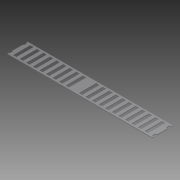
# Autodesk Inventor part: Wing
Saved by Autodesk Inventor 2013 (Build 170138000, 138)
## iProperties
Created: 2013-01-27
Part Number: Wing
Material: Polycarbonate, Clear
Document SubType Name: Modeling
Designer: Andrew Toennies
Density: 1.2 g/cm^3
Mass: 103.546 g
Surface Area: 686.087 cm^2
Volume: 86.2881 cm^3
Author: Andrew Toennies
Autodesk Inventor part; units mm, degrees
ref_plane "YZ Plane" through (0, 0, 0) normal (1, 0, 0) x (0, 1, 0)
ref_plane "XZ Plane" through (0, 0, 0) normal (0, 1, 0) x (-1, 0, 0)
ref_plane "XY Plane" through (0, 0, 0) normal (0, 0, 1) x (1, 0, 0)
sketch "Sketch1" plane through (0, 0, 0) normal (0, 1, 0) x (-1, 0, 0)
  line L0 (0, 0) -> (558.8, 0)
  line L1 (558.8, 0) -> (558.8, 79.375)
  line L2 (558.8, 79.375) -> (0, 79.375)
  line L3 (0, 79.375) -> (0, 0)
  dimension "d0" = 79.375
  dimension "d1" = 558.8
  constraints: 8 end point, 2 parallel, 1 horizontal, 1 perpendicular
  measures "d0" distance of L2.end L0.start
  measures "d1" distance of L1.end L2.end
extrude "Extrusion1" add sketch "Sketch1" along normal blind 3.175
sketch "Sketch3" plane through (-558.8, 0, 0) normal (-1, 0, 0) x (0, 0, 1)
  line L0 (0, 0) -> (79.375, 0) projected
  line L1 (79.375, 0) -> (79.375, 3.175) projected
  line L2 (0, 3.175) -> (79.375, 3.175) projected
  line L3 (0, 0) -> (0, 3.175) projected
  line L4 (73.025, 3.175) -> (73.025, 0)
  line L5 (60.325, 0) -> (60.325, 3.175)
  line L6 (19.05, 0) -> (19.05, 3.175)
  line L7 (6.35, 0) -> (6.35, 3.175)
  dimension "d4" = 12.7
  dimension "d5" = 6.35
  dimension "d6" = 12.7
  dimension "d7" = 6.35
  constraints: 8 end point, 8 point on line, 4 perpendicular
  measures "d4" distance between parallel lines of L5 L4
  measures "d5" distance between parallel lines of L1 L4
  measures "d6" distance between parallel lines of L6 L7
  measures "d7" distance between parallel lines of L3 L7
extrude "Extrusion2" cut sketch "Sketch3" against normal blind 3.175 contours L7 L2 L6 L0 | L5 L2 L4 L0
sketch "Sketch4" plane through (0, 0, 79.375) normal (1, 0, 0) x (0, 0, -1)
  line L0 (19.05, 3.175) -> (6.35, 3.175) projected
  line L1 (19.05, 0) -> (19.05, 3.175) projected
  line L2 (6.35, 0) -> (19.05, 0) projected
  line L3 (6.35, 3.175) -> (6.35, 0) projected
  line L4 (60.325, 3.175) -> (60.325, 0) projected
  line L5 (73.025, 3.175) -> (60.325, 3.175) projected
  line L6 (73.025, 0) -> (73.025, 3.175) projected
  line L7 (60.325, 0) -> (73.025, 0) projected
extrude "Extrusion3" cut sketch "Sketch4" against normal blind 6.35
sketch "Sketch5" plane through (0, 0, 0) normal (0, -1, 0) x (1, 0, 0)
  line L0 (-558.8, 79.375) -> (0, 79.375) projected
  line L1 (-558.8, 19.05) -> (-558.8, 60.325) projected
  line L2 (0, 0) -> (-558.8, 0) projected
  line L3 (-542.925, 73.025) -> (-542.925, 6.35)
  line L4 (-542.925, 6.35) -> (-530.225, 6.35)
  line L5 (-542.925, 73.025) -> (-530.225, 73.025)
  line L6 (-530.225, 73.025) -> (-530.225, 6.35)
  line L7 (-517.525, 73.025) -> (-517.525, 6.35)
  line L8 (-517.525, 6.35) -> (-504.825, 6.35)
  line L9 (-517.525, 73.025) -> (-504.825, 73.025)
  line L10 (-504.825, 73.025) -> (-504.825, 6.35)
  line L11 (-492.125, 73.025) -> (-492.125, 6.35)
  line L12 (-492.125, 6.35) -> (-479.425, 6.35)
  line L13 (-492.125, 73.025) -> (-479.425, 73.025)
  line L14 (-479.425, 73.025) -> (-479.425, 6.35)
  line L15 (-466.725, 73.025) -> (-466.725, 6.35)
  line L16 (-466.725, 6.35) -> (-454.025, 6.35)
  line L17 (-466.725, 73.025) -> (-454.025, 73.025)
  line L18 (-454.025, 73.025) -> (-454.025, 6.35)
  line L19 (-441.325, 73.025) -> (-441.325, 6.35)
  line L20 (-441.325, 6.35) -> (-428.625, 6.35)
  line L21 (-441.325, 73.025) -> (-428.625, 73.025)
  line L22 (-428.625, 73.025) -> (-428.625, 6.35)
  line L23 (-415.925, 73.025) -> (-415.925, 6.35)
  line L24 (-415.925, 6.35) -> (-403.225, 6.35)
  line L25 (-415.925, 73.025) -> (-403.225, 73.025)
  line L26 (-403.225, 73.025) -> (-403.225, 6.35)
  line L27 (-390.525, 73.025) -> (-390.525, 6.35)
  line L28 (-390.525, 6.35) -> (-377.825, 6.35)
  line L29 (-390.525, 73.025) -> (-377.825, 73.025)
  line L30 (-377.825, 73.025) -> (-377.825, 6.35)
  line L31 (-365.125, 73.025) -> (-365.125, 6.35)
  line L32 (-365.125, 6.35) -> (-352.425, 6.35)
  line L33 (-365.125, 73.025) -> (-352.425, 73.025)
  line L34 (-352.425, 73.025) -> (-352.425, 6.35)
  line L35 (-339.725, 73.025) -> (-339.725, 6.35)
  line L36 (-339.725, 6.35) -> (-327.025, 6.35)
  line L37 (-339.725, 73.025) -> (-327.025, 73.025)
  line L38 (-327.025, 73.025) -> (-327.025, 6.35)
  line L39 (-314.325, 73.025) -> (-314.325, 6.35)
  line L40 (-314.325, 6.35) -> (-301.625, 6.35)
  line L41 (-314.325, 73.025) -> (-301.625, 73.025)
  line L42 (-301.625, 73.025) -> (-301.625, 6.35)
  line L43 (-288.925, 73.025) -> (-288.925, 6.35)
  line L44 (-288.925, 6.35) -> (-276.225, 6.35)
  line L45 (-288.925, 73.025) -> (-276.225, 73.025)
  line L46 (-276.225, 73.025) -> (-276.225, 6.35)
  line L47 (-263.525, 73.025) -> (-263.525, 6.35)
  line L48 (-263.525, 6.35) -> (-250.825, 6.35)
  line L49 (-263.525, 73.025) -> (-250.825, 73.025)
  line L50 (-250.825, 73.025) -> (-250.825, 6.35)
  line L51 (-238.125, 73.025) -> (-238.125, 6.35)
  line L52 (-238.125, 6.35) -> (-225.425, 6.35)
  line L53 (-238.125, 73.025) -> (-225.425, 73.025)
  line L54 (-225.425, 73.025) -> (-225.425, 6.35)
  line L55 (-212.725, 73.025) -> (-212.725, 6.35)
  line L56 (-212.725, 6.35) -> (-200.025, 6.35)
  line L57 (-212.725, 73.025) -> (-200.025, 73.025)
  line L58 (-200.025, 73.025) -> (-200.025, 6.35)
  line L59 (-187.325, 73.025) -> (-187.325, 6.35)
  line L60 (-187.325, 6.35) -> (-174.625, 6.35)
  line L61 (-187.325, 73.025) -> (-174.625, 73.025)
  line L62 (-174.625, 73.025) -> (-174.625, 6.35)
  line L63 (-161.925, 73.025) -> (-161.925, 6.35)
  line L64 (-161.925, 6.35) -> (-149.225, 6.35)
  line L65 (-161.925, 73.025) -> (-149.225, 73.025)
  line L66 (-149.225, 73.025) -> (-149.225, 6.35)
  line L67 (-136.525, 73.025) -> (-136.525, 6.35)
  line L68 (-136.525, 6.35) -> (-123.825, 6.35)
  line L69 (-136.525, 73.025) -> (-123.825, 73.025)
  line L70 (-123.825, 73.025) -> (-123.825, 6.35)
  line L71 (-111.125, 73.025) -> (-111.125, 6.35)
  line L72 (-111.125, 6.35) -> (-98.425, 6.35)
  line L73 (-111.125, 73.025) -> (-98.425, 73.025)
  line L74 (-98.425, 73.025) -> (-98.425, 6.35)
  line L75 (-85.725, 73.025) -> (-85.725, 6.35)
  line L76 (-85.725, 6.35) -> (-73.025, 6.35)
  line L77 (-85.725, 73.025) -> (-73.025, 73.025)
  line L78 (-73.025, 73.025) -> (-73.025, 6.35)
  line L79 (-60.325, 73.025) -> (-60.325, 6.35)
  line L80 (-60.325, 6.35) -> (-47.625, 6.35)
  line L81 (-60.325, 73.025) -> (-47.625, 73.025)
  line L82 (-47.625, 73.025) -> (-47.625, 6.35)
  line L83 (-34.925, 73.025) -> (-34.925, 6.35)
  line L84 (-34.925, 6.35) -> (-22.225, 6.35)
  line L85 (-34.925, 73.025) -> (-22.225, 73.025)
  line L86 (-22.225, 73.025) -> (-22.225, 6.35)
  dimension "d12" = 12.7
  dimension "d14" = 15.875
  dimension "d15" = 6.35
  dimension "d16" = 6.35
  dimension "d19" = 25.4
  constraints: 168 end point, 2 parallel, 2 perpendicular, 1 horizontal, 160 other
  measures "d12" distance of L3.end L4.end
  measures "d14" distance between parallel lines of L1 L3
  measures "d15" distance between parallel lines of L0 L5
  measures "d16" distance between parallel lines of L2 L4
  measures "d19" distance of L5.end L10.start
extrude "Extrusion4" cut sketch "Sketch5" against normal blind 25.4 contours L5 L6 L4 L3 | L9 L10 L8 L7 | L13 L14 L12 L11 | L17 L18 L16 L15 | L21 L22 L20 L19 | L25 L26 L24 L23 | L29 L30 L28 L27 | L33 L34 L32 L31 | L37 L38 L36 L35 | L45 L46 L44 L43 | L49 L50 L48 L47 | L53 L54 L52 L51 | L57 L58 L56 L55 | L61 L62 L60 L59 | L65 L66 L64 L63 | L69 L70 L68 L67 | L73 L74 L72 L71 | L77 L78 L76 L75 | L81 L82 L80 L79 | L85 L86 L84 L83
body "Solid1"
